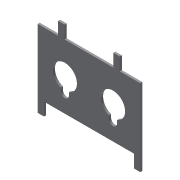
# Autodesk Inventor part: adaptplate
Saved by Autodesk Inventor 2022 (Build 260148000, 148)
## iProperties
Shininess: 64.0
Length Units: 11272
Angle Units: 11279
Time Units: 11290
Mass Units: 11286
Length Display Precision: 3
Angle Display Precision: 2
Created: 2002-05-03
Part Number: adaptplate
Document SubType Name: Modeling
Designer: Administrator
Density: 1 g/cm^3
Material: Generic
Appearance: Default
Density: 0.0
Volumn: 0.0
Area: 0.0
PropertySet Name: Model Information
Control State: 0
Master: False
Checked Out: False
Author: Administrator
Autodesk Inventor part; units mm, degrees
ref_plane "YZ Plane" through (0, 0, 0) normal (1, 0, 0) x (0, 1, 0)
ref_plane "XZ Plane" through (0, 0, 0) normal (0, 1, 0) x (-1, 0, 0)
ref_plane "XY Plane" through (0, 0, 0) normal (0, 0, 1) x (1, 0, 0)
sketch "Sketch1" plane through (0, 0, 0) normal (0, 0, 1) x (1, 0, 0)
  line L0 (-21.87, 21.3003) -> (-21.87, -9.1797)
  line L1 (-21.87, -9.1797) -> (-19.33, -9.1797)
  line L2 (-19.33, -9.1797) -> (-19.33, -4.0997)
  line L3 (-19.33, -4.0997) -> (16.23, -4.0997)
  line L4 (16.23, -4.0997) -> (16.23, -9.1797)
  line L5 (16.23, -9.1797) -> (18.77, -9.1797)
  line L6 (18.77, -9.1797) -> (18.77, 21.3003)
  line L7 (18.77, 21.3003) -> (10.6439, 21.3003)
  line L8 (10.6439, 21.3003) -> (10.6439, 26.3803)
  line L9 (10.6439, 26.3803) -> (8.1039, 26.3803)
  line L10 (8.1039, 26.3803) -> (8.1039, 21.3003)
  line L11 (8.1039, 21.3003) -> (-11.2039, 21.3003)
  line L12 (-11.2039, 21.3003) -> (-11.2039, 26.3803)
  line L13 (-11.2039, 26.3803) -> (-13.7439, 26.3803)
  line L14 (-13.7439, 26.3803) -> (-13.7439, 21.3003)
  line L15 (-13.7439, 21.3003) -> (-21.87, 21.3003)
  dimension "d0" = 40.64
  dimension "d1" = 25.4
  dimension "d2" = 5.08
  dimension "d3" = 2.54
  dimension "d5" = 5.08
  dimension "d18" = 2.54
  constraints: 32 end point, 13 parallel, 7 collinear, 1 perpendicular, 1 vertical
  measures "d0" distance of L5.end L0.end
  measures "d1" vertical distance of L0.start L2.end
  measures "d2" distance of L13.end L14.end
  measures "d3" distance of L12.end L13.end
  measures "d5" vertical distance of L2.end L0.end
  measures "d18" distance of L0.end L1.end
extrude "Extrusion1" add sketch "Sketch1" along normal blind 0.8255
sketch "Sketch2" plane through (0, 0, 0.8255) normal (0, 0, 1) x (1, 0, 0)
  line L0 (-13.7439, 21.3003) -> (-13.7439, 26.3803) projected
  arc A0 (-9.4748, 4.1012) -> (-12.6752, 4.1012) centre (-11.075, 8.6003) ccw
  line L1 (-12.6752, 4.1012) -> (-12.6752, 2.8853)
  arc A1 (-12.6752, 2.8853) -> (-9.4748, 2.8853) centre (-11.075, 2.8853) ccw
  line L2 (-9.4748, 2.8853) -> (-9.4748, 4.1012)
  line L3 (-21.87, -9.1797) -> (-21.87, 21.3003) projected
  point P0 (-19.33, -4.0997)
  dimension "d8" = 5.715
  dimension "d9" = 4.7752
  dimension "d10" = 1.6002
  dimension "d16" = 10.795
  dimension "d17" = 12.7
  constraints: 4 end point, 4 point on circle, 2 centre point, 2 parallel, 2 tangent, 1 vertical alignment
  measures "d8" distance of A1.centre A0.centre
  measures "d9" radius of A0
  measures "d10" radius of A1
  measures "d16" distance from line of A0.centre L3
  measures "d17" vertical distance of point (-19.33, -4.1) A0.centre
extrude "Extrusion2" cut sketch "Sketch2" against normal blind 0.8255
pattern_linear "Rectangular Pattern1" count 2 spacing 19.05 along (1, 0, 0) of "Extrusion2"
body "Solid1"
